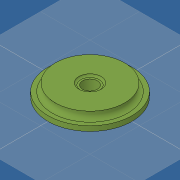
# Autodesk Inventor part: Unterdruckventil_Membran
Saved by Autodesk Inventor 2019 (Build 230136000, 136)
## iProperties
Created: 2020-09-01
Part Number: Unterdruckventil_Membran
Material: Generisch
Document SubType Name: Modeling
Designer: Stefan
Mass: 3.44375 g
Surface Area: 23.1606 cm^2
Volume: 3.44375 cm^3
Density: 1 g/cm^3
Appearance: Olivgrün
Author: Stefan
Autodesk Inventor part; units mm, degrees
ref_plane "YZ Plane" through (0, 0, 0) normal (1, 0, 0) x (0, 1, 0)
ref_plane "XZ Plane" through (0, 0, 0) normal (0, 1, 0) x (-1, 0, 0)
ref_plane "XY Plane" through (0, 0, 0) normal (0, 0, 1) x (1, 0, 0)
sketch "Skizze1" plane through (0, 0, 0) normal (0, 1, 0) x (-1, 0, 0)
  circle A0 centre (0, 0) radius 17
  circle A1 centre (0, 0) radius 3
  dimension "d6" = 34
  dimension "d12" = 6
  constraints: 2 centre point, 2 coincident
  measures "d6" diameter of A0
  measures "d12" diameter of A1
extrude "Extrusion1" add sketch "Skizze1" along normal blind 5
sketch "Skizze4" plane through (0, 0, 0) normal (0, 0, 1) x (1, 0, 0)
  line L0 (17, 5) -> (17, 0) projected
  line L1 (17, 0) -> (3, 0) projected
  line L2 (3, 0) -> (3, 5) projected
  line L3 (3, 5) -> (17, 5) projected
  line L4 (-17, 0) -> (-17, 5) projected
  line L5 (-17, 5) -> (-3, 5) projected
  line L6 (-3, 5) -> (-3, 0) projected
  line L7 (-3, 0) -> (-17, 0) projected
  line L8 (0, -0.6) -> (0, 3.6) projected
  line L9 (-14.0253, 5) -> (-17, 5)
  line L10 (-17, 5) -> (-17, 2)
  line L11 (-17, 2) -> (-15.25, 2)
  arc A0 (-15.25, 2) -> (-14.0253, 5) centre (-15.25, 3.75) ccw
  arc A1 (-4.5, 5) -> (-3.75, 4.25) centre (-3.75, 5) ccw
  line L12 (-4.5, 5) -> (-3, 5)
  line L13 (-3, 5) -> (-3, 4.25)
  line L14 (-3, 4.25) -> (-3.75, 4.25)
  point P0 (0, 0)
  dimension "d21" = 1.75
  dimension "d22" = 3
  dimension "d24" = 1.75
  dimension "d25" = 0.75
  dimension "d26" = 9
  constraints: 12 end point, 4 point on circle, 4 point on line, 2 centre point, 2 horizontal, 2 tangent, 1 collinear, 1 line through centre, 1 perpendicular
  measures "d21" radius of A0
  measures "d22" distance between parallel lines of L5 L11
  measures "d24" distance from line of L4 A0.centre
  measures "d25" distance between parallel lines of L12 L14
  measures "d26" diameter of L12.start L8
revolve "Umdrehung3" cut sketch "Skizze4" angle 360 about axis through (0, -10, 0) along (0, 1, 0) contours L4 L5 A0 L11 | L14 A1 L5 L6
